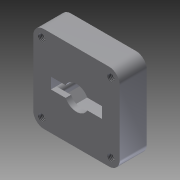
# Autodesk Inventor part: BD gearbox mount block 2
Saved by Autodesk Inventor 2012 (Build 160160000, 160)
## iProperties
Created: 2012-07-04
Part Number: BD gearbox mount block 2
Material: Default
Document SubType Name: Modeling
Designer: Bruce
Density: 1 g/cm^3
Author: Bruce
Autodesk Inventor part; units mm, degrees
ref_plane "YZ Plane" through (0, 0, 0) normal (1, 0, 0) x (0, 1, 0)
ref_plane "XZ Plane" through (0, 0, 0) normal (0, 1, 0) x (-1, 0, 0)
ref_plane "XY Plane" through (0, 0, 0) normal (0, 0, 1) x (1, 0, 0)
sketch "Sketch1" plane through (0, 0, 0) normal (0, 0, 1) x (1, 0, 0)
  line L0 (-13, 12) -> (13, 12)
  line L1 (13, 12) -> (13, -12)
  line L2 (13, -12) -> (-13, -12)
  line L3 (-13, -12) -> (-13, 12)
  line L4 (-13, 3.25) -> (-15, 3.25)
  line L5 (-15, 3.25) -> (-15, -3.25)
  line L6 (-15, -3.25) -> (-13, -3.25)
  line L7 (-13, -3.25) -> (-13, 3.25)
  line L8 (13, 3.25) -> (15, 3.25)
  line L9 (15, 3.25) -> (15, -3.25)
  line L10 (15, -3.25) -> (13, -3.25)
  line L11 (13, -3.25) -> (13, 3.25)
  line L12 (-25.4, 25.4) -> (25.4, 25.4)
  line L13 (25.4, 25.4) -> (25.4, -25.4)
  line L14 (25.4, -25.4) -> (-25.4, -25.4)
  line L15 (-25.4, -25.4) -> (-25.4, 25.4)
  circle A0 centre (0, 0) radius 7.1437
  circle A1 centre (-3, 12) radius 1.5
  line L16 (-13, 8) -> (-9, 12)
  line L17 (9, 12) -> (13, 8)
  line L18 (13, -8) -> (9, -12)
  line L19 (-13, -8) -> (-9, -12)
  line L20 (-13, 3.25) -> (13, 3.25)
  line L21 (13, -3.25) -> (-13, -3.25)
  point P0 (-14, 3.25)
  point P1 (14, 3.25)
  point P2 (-14, -3.25)
  point P3 (14, -3.25)
  point P4 (-20.32, 20.32)
  point P5 (20.32, 20.32)
  point P6 (20.32, -20.32)
  point P7 (-20.32, -20.32)
  dimension "d0" = 24
  dimension "d1" = 12
  dimension "d2" = 26
  dimension "d3" = 13
  dimension "d4" = 2
  dimension "d5" = 6.5
  dimension "d6" = 3.25
  dimension "d7" = 2
  dimension "d8" = 14.2875
  dimension "d9" = 50.8
  dimension "d10" = 25.4
  dimension "d11" = 50.8
  dimension "d12" = 25.4
  dimension "d13" = 3
  dimension "d14" = 10
  dimension "d15" = 4
  dimension "d16" = 4
  dimension "d17" = 4
  dimension "d18" = 4
  dimension "d19" = 4
  dimension "d20" = 5.08
  dimension "d21" = 5.08
  dimension "d22" = 5.08
  dimension "d23" = 5.08
  dimension "d34" = 40.64
  dimension "d35" = 40.64
  constraints: 44 end point, 10 point on line, 9 parallel, 8 perpendicular, 4 horizontal, 4 horizontal alignment, 4 midpoint, 2 centre point, 2 vertical alignment, 1 coincident, 1 collinear
  measures "d0" distance between parallel lines of L2 L0
  measures "d1" distance from line of L0 point (0, 0)
  measures "d2" distance of L1.end L2.end
  measures "d3" distance from line of L1 point (0, 0)
  measures "d4" distance between parallel lines of L3 L5
  measures "d5" distance of L4.end L5.end
  measures "d6" distance from line of L4 point (0, 0)
  measures "d7" distance between parallel lines of L11 L9
  measures "d8" diameter of A0
  measures "d9" distance of L12.end L13.end
  measures "d10" distance from line of L12 point (0, 0)
  measures "d11" distance of L13.end L14.end
  measures "d12" distance from line of L13 point (0, 0)
  measures "d13" diameter of A1
  measures "d14" distance from line of A1.centre L3
  measures "d15" distance of L0.start L16.end
  measures "d16" distance of L16.start L0.start
  measures "d17" distance from line of L17.start L1
  measures "d18" distance of L2.end L19.start
  measures "d19" distance of L1.end L18.start
  measures "d20" distance from line of point (-20.32, 20.32) L12
  measures "d21" distance from line of L15 point (-20.32, 20.32)
  measures "d22" distance from line of L14 point (-20.32, -20.32)
  measures "d23" distance from line of point (20.32, 20.32) L13
  measures "d34" distance of point (20.32, 20.32) point (-20.32, 20.32)
  measures "d35" distance of point (-20.32, 20.32) point (-20.32, -20.32)
extrude "Extrusion1" add sketch "Sketch1" against normal blind 12.7 contours L0 L16 L3 | L0 L1 L17 | L19 L2 L3 | L18 L1 L2 | L12 L13 L14 L15
fillet "Fillet1" radius 3.175 4 edges at (-13, -3.25, -6.35) (-13, 3.25, -6.35) (13, 3.25, -6.35) (13, -3.25, -6.35)
extrude "Extrusion2" add sketch "Sketch1" along normal blind 3.175 contours L0 L16 L3 | L0 A1 L17 L1 L20 A0 L3 L16 | A1 L0 | L0 A1 | L21 A0 L1 L18 L2 L19 L3 | L0 L1 L17 | L19 L2 L3 | L18 L1 L2 | L12 L13 L14 L15
hole "Hole1" at (-20.32, 20.32, 0) at (20.32, 20.32, 0) at (20.32, -20.32, 0) at (-20.32, -20.32, 0) direction (0, 0, -1) diameter 4.1656 end through all
thread "Thread1" size "10-32 UNF" class "2B" standard "ANSI Unified Screw Threads" full length
thread "Thread2" size "10-32 UNF" class "2B" standard "ANSI Unified Screw Threads" full length
thread "Thread3" size "10-32 UNF" class "2B" standard "ANSI Unified Screw Threads" full length
thread "Thread4" size "10-32 UNF" class "2B" standard "ANSI Unified Screw Threads" full length
hole "Hole2" at (20.32, 20.32, 0) at (-20.32, 20.32, 0) at (-20.32, -20.32, 0) at (20.32, -20.32, 0) direction (0, 0, 1) diameter 4.1656 end through all
fillet "Fillet2" radius 6.35 4 edges at (25.4, 25.4, -4.7625) (-25.4, 25.4, -4.7625) (-25.4, -25.4, -4.7625) (25.4, -25.4, -4.7625)
equation "\"d1\" = 0.5 * d0"
equation "\"d3\" = 0.5 * d2"
equation "\"d6\" = 0.5 * d5"
equation "\"d7\" = d4"
equation "\"d10\" = 0.5 * d9"
equation "\"d12\" = 0.5 * d11"
equation "\"d16\" = d15"
equation "\"d17\" = d15"
equation "\"d18\" = d15"
equation "\"d19\" = d15"
equation "\"d22\" = d21"
equation "\"d23\" = d21"
body "Solid1"
